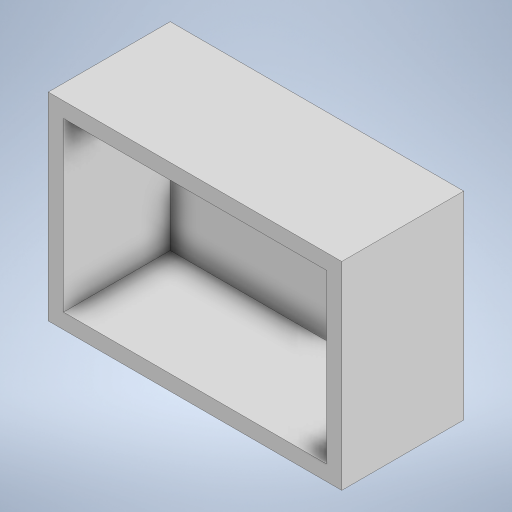
# Autodesk Inventor part: Box
Saved by Autodesk Inventor 2023 (Build 270158000, 158)
## iProperties
Created: 2023-04-23
Part Number: Box
Material: Generic
Document SubType Name: Modeling
Designer: ringl
Density: 1 g/cm^3
Appearance: Default
Author: ringl
Autodesk Inventor part; units mm, degrees
ref_plane "YZ Plane" through (0, 0, 0) normal (1, 0, 0) x (0, 1, 0)
ref_plane "XZ Plane" through (0, 0, 0) normal (0, 1, 0) x (-1, 0, 0)
ref_plane "XY Plane" through (0, 0, 0) normal (0, 0, 1) x (1, 0, 0)
sketch "Sketch1" plane through (0, 0, 0) normal (0, 0, 1) x (1, 0, 0)
  line L0 (0, 0) -> (38.5, 0)
  line L1 (38.5, 0) -> (38.5, 26)
  line L2 (38.5, 26) -> (0, 26)
  line L3 (0, 26) -> (0, 0)
  dimension "d0" = 38.5
  dimension "d1" = 26
  constraints: 8 end point, 2 parallel, 1 horizontal, 1 perpendicular
  measures "d0" distance of L2.end L1.end
  measures "d1" distance of L0.end L1.end
extrude "Extrusion1" add sketch "Sketch1" along normal blind 16
sketch "Sketch2" plane through (0, 0, 16) normal (0, 0, 1) x (1, 0, 0)
  line L0 (2, 2) -> (36.5, 2)
  line L1 (36.5, 2) -> (36.5, 24)
  line L2 (36.5, 24) -> (2, 24)
  line L3 (2, 24) -> (2, 2)
  line L4 (38.5, 0) -> (38.5, 26) projected
  line L5 (38.5, 26) -> (0, 26) projected
  line L6 (0, 0) -> (38.5, 0) projected
  line L7 (0, 26) -> (0, 0) projected
  point P0 (36.5, 13)
  dimension "d4" = 2
  dimension "d5" = 2
  dimension "d6" = 2
  dimension "d7" = 2
  constraints: 8 end point, 2 parallel, 1 horizontal, 1 midpoint, 1 perpendicular
  measures "d4" distance from line of L4 point (36.5, 13)
  measures "d5" distance between parallel lines of L5 L2
  measures "d6" distance between parallel lines of L6 L0
  measures "d7" distance between parallel lines of L7 L3
extrude "Extrusion2" cut sketch "Sketch2" against normal blind 14 contours L3 L2 L1 L0
body "Solid1"
